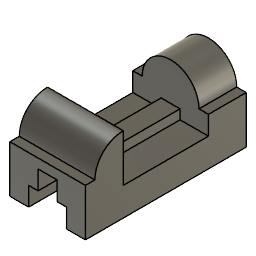
RoboconT1(Part-2) (Autodesk Fusion 360 design; units mm, degrees)
part number: 2026-03-05-11-47-04-601
Autodesk Fusion 360 part; units mm, degrees
note: some values were not read from the file. Set by a fixed rule: which sketch regions a step uses.
sketch "Sketch1" plane through (0, 0, 0) normal (1, 0, 0) x (0, 1, 0)
  line L0 (-42.5, 0) -> (42.5, 0)
  line L1 (-42.5, 0) -> (-42.5, 25)
  line L2 (-42.5, 25) -> (-37.5, 25)
  arc A0 (-22.5, 40) -> (-37.5, 25) centre (-22.5, 25) ccw
  line L3 (-22.5, 40) -> (-22.5, 15)
  line L4 (-22.5, 15) -> (22.5, 15)
  line L5 (22.5, 15) -> (22.5, 25)
  line L6 (42.5, 0) -> (42.5, 25)
  line L7 (42.5, 25) -> (22.5, 25)
  constraint perpendicular L0 L1
  constraint perpendicular L1 L2
  constraint perpendicular L0 L3
  constraint perpendicular L3 L4
  constraint perpendicular L4 L5
  constraint perpendicular L0 L6
  constraint perpendicular L5 L7
extrude "Extrude2" add sketch "Sketch1" along normal mid plane 40 makes body 1
sketch "Sketch2" plane through (0, 22.5, 0) normal (0, -1, 0) x (1, 0, 0)
  line L0 (-20, 15) -> (20, 15)
  line L1 (20, 15) -> (20, 25)
  line L2 (-20, 25) -> (-20, 15)
  arc A0 (15, 25) -> (-15, 25) centre (0, 25) ccw
  line L3 (20, 25) -> (-20, 25)
extrude "Extrude3" add sketch "Sketch2" against normal blind 20 contours A0 L3 bodies 1
sketch "Sketch3" plane through (0, -42.5, 0) normal (0, -1, 0) x (1, 0, 0)
  line L0 (-20, 0) -> (20, 0)
  line L1 (20, 0) -> (20, 25)
  line L2 (20, 25) -> (-20, 25)
  line L3 (-20, 25) -> (-20, 0)
  line L4 (-10, 0) -> (10, 0)
  line L5 (-10, 0) -> (-10, 10)
  line L6 (10, 0) -> (10, 10)
  line L7 (-10, 10) -> (-5, 10)
  line L8 (-5, 10) -> (-5, 20)
  line L9 (-5, 20) -> (5, 20)
  line L10 (5, 20) -> (5, 10)
  line L11 (5, 10) -> (10, 10)
  constraint coincident L0 L4.start
  constraint coincident L0 L4.end
  constraint perpendicular L0 L5
  constraint perpendicular L4 L6
  constraint perpendicular L5 L7
  constraint perpendicular L4 L8
  constraint perpendicular L8 L9
  constraint perpendicular L9 L10
  constraint perpendicular L10 L11
extrude "Extrude4" cut sketch "Sketch3" against normal blind 85 contours L0 L4 L5 L6 L7 L8 L9 L10 L11 bodies 1
sketch "Sketch4" plane through (0, 0, 15) normal (0, 0, 1) x (-1, 0, 0)
  line L0 (-5, -22.5) -> (-5, 22.5)
  line L1 (-5, 22.5) -> (-20, 22.5)
  line L2 (-20, 22.5) -> (-20, -22.5)
  line L3 (-20, -22.5) -> (-5, -22.5)
  line L4 (-5, -22.5) -> (5, -22.5)
  line L5 (5, -22.5) -> (5, 22.5)
  line L6 (5, 22.5) -> (-5, 22.5)
  constraint coincident L0.start L3.end
  constraint perpendicular L0 L4
  constraint perpendicular L4 L5
  constraint coincident L0.end L1.start
extrude "Extrude5" add sketch "Sketch4" along normal blind 5 separate body contours L0 L4 L5 L6 makes body 2
named bodies: "Body1", "Body2"
